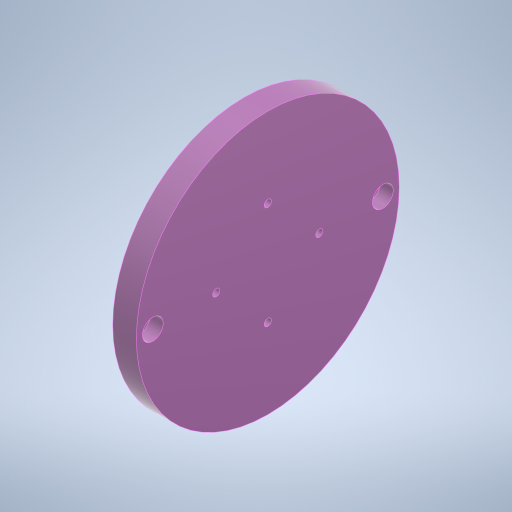
# Autodesk Inventor part: laboratory_equipment-GIM3505-8
Saved by Autodesk Inventor 2024 (Build 280153000, 153)
## iProperties
Created: 2025-04-23
Part Number: laboratory_equipment-GIM3505-8
Material: ABS プラスチック
Document SubType Name: Modeling
Designer: 1412z
Density: 1.06 g/cm^3
Appearance: 滑らか - 紫
Author: 1412z
Autodesk Inventor part; units mm, degrees
ref_plane "YZ Plane" through (0, 0, 0) normal (1, 0, 0) x (0, 1, 0)
ref_plane "XZ Plane" through (0, 0, 0) normal (0, 1, 0) x (-1, 0, 0)
ref_plane "XY Plane" through (0, 0, 0) normal (0, 0, 1) x (1, 0, 0)
sketch "スケッチ1" plane through (0, 0, 0) normal (1, 0, 0) x (0, 1, 0)
  circle A0 centre (0, 0) radius 19.6
  circle A1 centre (0, 19.6) radius 1.4
  circle A2 centre (-19.6, 0) radius 1.4
  circle A3 centre (0, -19.6) radius 1.4
  circle A4 centre (19.6, 0) radius 1.4
  circle A5 centre (0, 0) radius 50
  dimension "d0" = 39.2
  dimension "d1" = 2.8
  dimension "d4" = 360
  dimension "d6" = 100
  constraints: 5 centre point, 2 coincident, 1 vertical alignment, 11 other
  measures "d1" diameter of A1
  measures "d6" diameter of A5
extrude "押し出し1" add sketch "スケッチ1" along normal blind 2 contours A4 A0 A3 A2 A1 | A5
sketch "スケッチ2" plane through (0, 0, 0) normal (-1, 0, 0) x (0, 0, 1)
  circle A0 centre (0, 0) radius 50
  circle A1 centre (0, 0) radius 37.5
  dimension "d9" = 75
  constraints: 2 centre point, 2 coincident
  measures "d9" diameter of A1
extrude "押し出し2" add sketch "スケッチ2" along normal blind 7
sketch "スケッチ3" plane through (2, 0, 0) normal (1, 0, 0) x (0, 0, -1)
  circle A0 centre (0, 0) radius 43.75
  circle A1 centre (-43.75, 0) radius 2.25
  circle A2 centre (43.75, 0) radius 2.25
  dimension "d12" = 87.5
  dimension "d13" = 4.5
  dimension "d14" = 4.5
  constraints: 3 centre point, 2 point on circle, 1 coincident
  measures "d12" diameter of A0
  measures "d13" diameter of A1
  measures "d14" diameter of A2
extrude "押し出し3" cut sketch "スケッチ3" against normal blind 10 contours A0 A2 | A0 A2 | A1 A0 | A0 A1
sketch "スケッチ4" plane through (2, 0, 0) normal (1, 0, 0) x (0, 0, -1)
  circle A0 centre (-43.75, 0) radius 2.25 projected
  circle A1 centre (-43.75, 0) radius 4
  circle A2 centre (43.75, 0) radius 2.25 projected
  circle A3 centre (43.75, 0) radius 4
  point P0 (0, 0)
  dimension "d17" = 8
  dimension "d18" = 8
  constraints: 2 centre point, 2 coincident
  measures "d17" diameter of A1
  measures "d18" diameter of A3
extrude "押し出し4" cut sketch "スケッチ4" against normal blind 5
